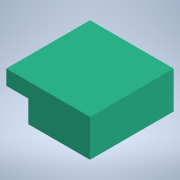
# Autodesk Inventor part: Intake
Saved by Autodesk Inventor 2022.3 (Build 263350000, 350)
## iProperties
Created: 2023-02-06
Part Number: Intake
Material: Generic
Document SubType Name: Modeling
Designer: lbmcgill42
Density: 1 g/cm^3
Appearance: Default
Author: lbmcgill42
Autodesk Inventor part; units mm, degrees
ref_plane "YZ Plane" through (0, 0, 0) normal (1, 0, 0) x (0, 1, 0)
ref_plane "XZ Plane" through (0, 0, 0) normal (0, 1, 0) x (-1, 0, 0)
ref_plane "XY Plane" through (0, 0, 0) normal (0, 0, 1) x (1, 0, 0)
sketch "Sketch1" plane through (0, 0, 0) normal (0, 1, 0) x (-1, 0, 0)
  line L0 (80.2529, 101.9539) -> (-206.7671, 101.9539)
  line L1 (-206.7671, 101.9539) -> (-206.7671, -185.0661)
  line L2 (-206.7671, -185.0661) -> (80.2529, -185.0661)
  line L3 (80.2529, -185.0661) -> (80.2529, 101.9539)
  point P0 (0, 0)
  dimension "d0" = 287.02
  dimension "d1" = 287.02
  constraints: 8 end point, 2 parallel, 1 horizontal, 1 perpendicular
  measures "d0" distance of L2.end L0.start
  measures "d1" distance of L0.start L0.end
extrude "Extrusion1" add sketch "Sketch1" along normal blind 127
sketch "Sketch2" plane through (0, 0, 0) normal (0, -1, 0) x (1, 0, 0)
  line L0 (-80.2529, 101.9539) -> (206.7671, 101.9539) projected
  line L1 (206.7671, -185.0661) -> (-80.2529, -185.0661) projected
  line L2 (-80.2529, 101.9539) -> (-4.0529, 101.9539)
  line L3 (-4.0529, 101.9539) -> (-4.0529, -185.0661)
  line L4 (-4.0529, -185.0661) -> (-80.2529, -185.0661)
  line L5 (-80.2529, -185.0661) -> (-80.2529, 101.9539)
  point P0 (0, 0)
  dimension "d4" = 76.2
  constraints: 8 end point, 2 parallel, 1 horizontal, 1 perpendicular, 1 point on line
  measures "d4" distance of L3.end L4.end
extrude "Extrusion2" cut sketch "Sketch2" against normal blind 76.2
body "Solid1"
